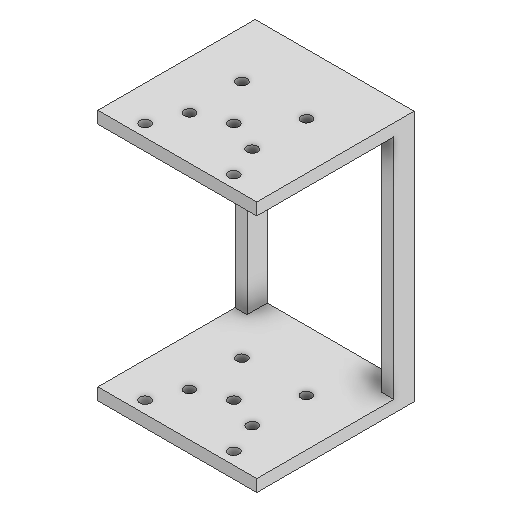
# Autodesk Inventor part: ARM_1 SKETCH
Saved by Autodesk Inventor 2025.3 (Build 293356030, 356C)
## iProperties
Created: 2025-09-30
Part Number: ARM_1 SKETCH
Material: 일반
Document SubType Name: Modeling
Designer: joseph
Density: 1 g/cm^3
Appearance: 기본값
Author: joseph
Autodesk Inventor part; units mm, degrees
ref_plane "YZ Plane" through (0, 0, 0) normal (1, 0, 0) x (0, 1, 0)
ref_plane "XZ Plane" through (0, 0, 0) normal (0, 1, 0) x (-1, 0, 0)
ref_plane "XY Plane" through (0, 0, 0) normal (0, 0, 1) x (1, 0, 0)
sketch "스케치1" plane through (0, 0, 0) normal (0, 0, 1) x (1, 0, 0)
  line L0 (-16.7, 28.2) -> (16.7, 28.2)
  line L1 (16.7, 28.2) -> (16.7, -28.2)
  line L2 (16.7, -28.2) -> (-16.7, -28.2)
  line L3 (-16.7, -28.2) -> (-16.7, 28.2)
  line L4 (19.7, -31.2) -> (19.7, 31.2)
  line L5 (19.7, 31.2) -> (-19.7, 31.2)
  line L6 (-19.7, 31.2) -> (-19.7, -31.2)
  line L7 (-19.7, -31.2) -> (19.7, -31.2)
  point P0 (0, 0)
  point P1 (-16.7, 0)
  point P2 (0, 28.2)
  dimension "d0" = 33.4
  dimension "d1" = 56.4
  dimension "d2" = 3
  constraints: 16 end point, 4 parallel, 2 midpoint, 2 perpendicular, 1 horizontal, 1 horizontal alignment, 1 vertical alignment, 3 other
  measures "d0" distance of L1.end L2.end
  measures "d1" distance of L0.end L1.end
  measures "d2" distance between parallel lines of L1 L4
extrude "돌출1" add sketch "스케치1" along normal blind 5
sketch "스케치3" plane through (-19.7, -31.2, 0) normal (0, -1, 0) x (1, 0, 0)
  line L0 (39.4, 0) -> (0, 0) projected
  line L1 (0, 0) -> (39.4, 0)
  line L2 (39.4, 0) -> (39.4, 39)
  line L3 (39.4, 39) -> (0, 39)
  line L4 (0, 39) -> (0, 0)
  line L5 (19.7, 39) -> (19.7, 0) construction
  line L6 (0, 36) -> (39.4, 36) construction
  circle A0 centre (19.7, 36) radius 11 construction
  circle A1 centre (8.7, 36) radius 1.3
  circle A2 centre (11.9218, 28.2218) radius 1.3
  circle A3 centre (19.7, 25) radius 1.3
  circle A4 centre (27.4782, 28.2218) radius 1.3
  circle A5 centre (30.7, 36) radius 1.3
  line L7 (0, 15) -> (39.4, 15) construction
  circle A6 centre (11.7, 15) radius 1.3
  circle A7 centre (27.7, 15) radius 1.3
  point P0 (39.4, 0)
  dimension "d9" = 22
  dimension "d5" = 39
  dimension "d8" = 3
  dimension "d10" = 2.6
  dimension "d13" = 180
  dimension "d15" = 24
  dimension "d16" = 2.6
  dimension "d17" = 2.6
  dimension "d18" = 8
  dimension "d19" = 8
  constraints: 14 end point, 7 centre point, 7 point on line, 3 perpendicular, 2 midpoint, 2 parallel, 1 horizontal, 1 horizontal alignment, 1 vertical, 11 other
  measures "d5" distance of L2.end L1.end
  measures "d8" distance between parallel lines of L3 L6
  measures "d10" diameter of A1
  measures "d15" distance between parallel lines of L3 L7
  measures "d16" diameter of A6
  measures "d17" diameter of A7
  measures "d18" distance from line of L5 A7.centre
  measures "d19" distance from line of L5 A6.centre
extrude "돌출2" add sketch "스케치3" against normal blind 3
mirror "미러1" about plane through (0, 0, 0) normal (0, 1, 0)
